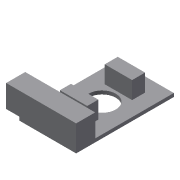
# Autodesk Inventor part: LG_CRD_8521B_Base
Saved by Autodesk Inventor 2019 (Build 230136000, 136)
## iProperties
Created: 2019-06-12
Part Number: LG_CRD_8521B_Base
Material: Generic
Document SubType Name: Modeling
Designer: diederichbenedict
Density: 1 g/cm^3
Appearance: Default
Author: diederichbenedict
Autodesk Inventor part; units mm, degrees
ref_plane "YZ Plane" through (0, 0, 0) normal (1, 0, 0) x (0, 1, 0)
ref_plane "XZ Plane" through (0, 0, 0) normal (0, 1, 0) x (-1, 0, 0)
ref_plane "XY Plane" through (0, 0, 0) normal (0, 0, 1) x (1, 0, 0)
sketch "Sketch1" plane through (0, 0, 0) normal (0, 1, 0) x (-1, 0, 0)
  line L0 (0, 0) -> (16.4, 0)
  line L1 (16.4, 0) -> (16.4, -28.2)
  line L2 (16.4, -28.2) -> (0, -28.2)
  line L3 (0, -28.2) -> (0, 0)
  dimension "d0" = 16.4
  dimension "d1" = 28.2
  constraints: 8 end point, 2 parallel, 1 horizontal, 1 perpendicular
  measures "d0" distance of L1.end L2.end
  measures "d1" distance of L0.end L1.end
extrude "Extrusion1" add sketch "Sketch1" along normal blind 1
sketch "Sketch2" plane through (0, 1, 0) normal (0, 1, 0) x (1, 0, 0)
  circle A0 centre (-8.2, 6) radius 0.5
  circle A1 centre (-8.2, 25.5) radius 0.5
  line L0 (-16.4, 0) -> (0, 0) projected
  line L1 (-16.4, 28.2) -> (-16.4, 0) projected
  circle A2 centre (-8.2, 15.7) radius 3.9462
  dimension "d4" = 1
  dimension "d5" = 1
  dimension "d6" = 6
  dimension "d7" = 19.5
  dimension "d8" = 8.2
  dimension "d9" = 8.2
  dimension "d10" = 9.7
  dimension "d11" = 9.8
  constraints: 3 centre point
  measures "d4" diameter of A0
  measures "d5" diameter of A1
  measures "d6" distance from line of A0.centre L0
  measures "d7" distance of A1.centre A0.centre
  measures "d8" distance from line of A0.centre L1
  measures "d9" distance from line of A1.centre L1
  measures "d10" distance of A2.centre A0.centre
  measures "d11" distance of A2.centre A1.centre
extrude "Extrusion2" cut sketch "Sketch2" against normal blind 1
sketch "Sketch3" plane through (0, 1, 0) normal (0, 1, 0) x (1, 0, 0)
  line L0 (0, 0) -> (-20.2, 0)
  line L1 (-20.2, 0) -> (-20.2, 5.5)
  line L2 (-20.2, 5.5) -> (0, 5.5)
  line L3 (0, 5.5) -> (0, 0)
  dimension "d14" = 20.2
  dimension "d15" = 5.5
  constraints: 8 end point, 2 parallel, 1 horizontal, 1 perpendicular
  measures "d14" distance of L1.end L2.end
  measures "d15" distance of L0.end L1.end
extrude "Extrusion3" add sketch "Sketch3" along normal blind 6.5
sketch "Sketch4" plane through (0, 1, 0) normal (0, 1, 0) x (1, 0, 0)
  line L0 (-8.2, 5.5) -> (0, 5.5) projected
  line L1 (0, 5.5) -> (0, 28.2) projected
  line L2 (0, 28.2) -> (-16.4, 28.2) projected
  line L3 (-16.4, 28.2) -> (-16.4, 5.5) projected
  line L4 (-16.4, 5.5) -> (-8.2, 5.5) projected
  circle A0 centre (-8.2, 6) radius 0.5 projected
  circle A1 centre (-8.2, 25.5) radius 0.5 projected
  circle A2 centre (-8.2, 15.7) radius 3.9462 projected
  line L5 (-12.1462, 7.4563) -> (-4.2538, 7.4563)
  line L6 (-4.2538, 7.4563) -> (-4.2538, 10.6519)
  line L7 (-4.2538, 10.6519) -> (-12.1462, 10.6519)
  line L8 (-12.1462, 10.6519) -> (-12.1462, 7.4563)
  line L9 (-12.1462, 24.1585) -> (-4.2538, 24.1585)
  line L10 (-4.2538, 24.1585) -> (-4.2538, 20.409)
  line L11 (-4.2538, 20.409) -> (-12.1462, 20.409)
  line L12 (-12.1462, 20.409) -> (-12.1462, 24.1585)
  point P0 (0, 0)
  constraints: 16 end point, 4 parallel, 2 horizontal, 2 perpendicular, 2 point on line, 1 vertical alignment
extrude "Extrusion4" add sketch "Sketch4" along normal blind 5 contours L8 L7 L6 L5 | L9 L10 L11 L12
body "Solid1"
